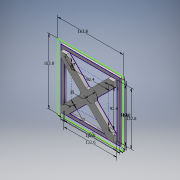
# Autodesk Inventor part: Lifting Motor Platform
Saved by Autodesk Inventor 2016 (Build 200138000, 138)
## iProperties
Created: 2016-03-08
Part Number: Lifting Motor Platform
Material: Generic
Document SubType Name: Modeling
Designer: Kenneth Daniel
Density: 1 g/cm^3
Appearance: Default
Author: Kenneth Daniel
Autodesk Inventor part; units mm, degrees
note: some values were not read from the file. Chosen so that the rebuilt part matches the saved one: sketch regions of "Extrusion5".
ref_plane "YZ Plane" through (0, 0, 0) normal (1, 0, 0) x (0, 1, 0)
ref_plane "XZ Plane" through (0, 0, 0) normal (0, 1, 0) x (-1, 0, 0)
ref_plane "XY Plane" through (0, 0, 0) normal (0, 0, 1) x (1, 0, 0)
sketch "Sketch1" plane through (0, 0, 0) normal (0, 1, 0) x (-1, 0, 0)
  line L0 (-81.5, 81.5) -> (81.5, -81.5) construction
  line L1 (-81.5, -81.5) -> (81.5, 81.5) construction
  line L2 (-66.3, 66.3) -> (66.3, -66.3) construction
  line L3 (-66.3, -66.3) -> (66.3, 66.3) construction
  line L4 (-81.9, 81.9) -> (-81.9, -81.9)
  line L5 (-81.9, -81.9) -> (81.9, -81.9)
  line L6 (81.9, -81.9) -> (81.9, 81.9)
  line L7 (81.9, 81.9) -> (-81.9, 81.9)
  line L8 (-66.1, 66.1) -> (-66.1, -66.1)
  line L9 (-66.1, -66.1) -> (66.1, -66.1)
  line L10 (66.1, -66.1) -> (66.1, 66.1)
  line L11 (66.1, 66.1) -> (-66.1, 66.1)
  line L12 (-66.1, 66.1) -> (66.1, -66.1) construction
  line L13 (-66.1, -66.1) -> (66.1, 66.1) construction
  line L14 (66.1, 51.9579) -> (17.2261, 3.084)
  line L15 (51.9579, 66.1) -> (3.084, 17.2261)
  line L16 (66.1, -51.9579) -> (14.1421, 0) construction
  line L17 (50.106, -64.2481) -> (3.084, -17.2261)
  arc A0 (-17.2261, -3.084) -> (-3.084, -17.2261) centre (0, 0) ccw
  arc A1 (-17.2261, 3.084) -> (-17.2261, -3.084) centre (0, 0) ccw
  line L18 (-14.1421, 0) -> (-17.2261, -3.084) construction
  line L19 (-3.084, 17.2261) -> (-51.9579, 66.1)
  line L20 (3.084, 17.2261) -> (0, 14.1421) construction
  line L21 (0, 14.1421) -> (-14.1421, 0) construction
  line L22 (14.1421, 0) -> (-3.084, 17.2261) construction
  arc A2 (17.2261, 3.084) -> (-17.2261, 3.084) centre (0, 0) ccw
  arc A3 (17.2261, -3.084) -> (17.2261, 3.084) centre (0, 0) ccw
  arc A4 (-3.084, -17.2261) -> (17.2261, -3.084) centre (0, 0) ccw
  line L23 (3.084, -17.2261) -> (0, -14.1421) construction
  line L24 (0, -14.1421) -> (-14.1421, 0) construction
  line L25 (17.2261, 3.084) -> (-3.084, -17.2261) construction
  line L26 (-3.084, -17.2261) -> (-51.9579, -66.1)
  line L27 (-17.2261, -3.084) -> (-66.1, -51.9579)
  line L28 (-17.2261, 3.084) -> (-64.2481, 50.106)
  line L29 (-14.1421, 0) -> (-17.2261, 3.084) construction
  line L30 (17.2261, -3.084) -> (66.1, -51.9579)
  line L31 (50.106, -64.2481) -> (51.9579, -66.1)
  line L32 (-64.2481, 50.106) -> (-66.1, 51.9579)
  line L33 (46.2, 46.2) -> (-46.2, 46.2) construction
  line L34 (-46.2, 46.2) -> (-46.2, -46.2) construction
  line L35 (-46.2, -46.2) -> (46.2, -46.2) construction
  line L36 (46.2, -46.2) -> (46.2, 46.2) construction
  line L37 (46.2, 46.2) -> (-46.2, -46.2) construction
  line L38 (-46.2, 46.2) -> (46.2, -46.2) construction
  circle A5 centre (46.2, -46.2) radius 1
  circle A6 centre (-46.2, -46.2) radius 1
  circle A7 centre (-46.2, 46.2) radius 1
  circle A8 centre (46.2, 46.2) radius 1
  line L39 (51.9579, 66.1) -> (66.1, 51.9579)
  line L40 (66.1, -51.9579) -> (51.9579, -66.1)
  line L41 (-51.9579, -66.1) -> (-66.1, -51.9579)
  line L42 (-66.1, 51.9579) -> (-51.9579, 66.1)
  line L43 (-74, 74) -> (-74, -74)
  line L44 (-74, -74) -> (74, -74)
  line L45 (74, -74) -> (74, 74)
  line L46 (74, 74) -> (-74, 74)
  line L47 (-74, 74) -> (74, -74) construction
  line L48 (-74, -74) -> (74, 74) construction
  dimension "d0" = 163
  dimension "d1" = 163
  dimension "d2" = 132.6
  dimension "d3" = 132.6
  dimension "d5" = 163.8
  dimension "d6" = 163.8
  dimension "d7" = 132.2
  dimension "d8" = 132.2
  dimension "d9" = 20
  dimension "d10" = 20
  dimension "d11" = 35
  dimension "d12" = 92.4
  dimension "d13" = 92.4
  dimension "d14" = 2
  dimension "d15" = 2
  dimension "d16" = 2
  dimension "d17" = 2
  dimension "d28" = 148
  dimension "d29" = 148
  constraints: 98 end point, 41 parallel, 23 point on line, 15 point on circle, 10 midpoint, 9 centre point, 7 perpendicular, 5 coincident, 2 vertical, 1 collinear, 1 horizontal, 2 other
  measures "d0" distance of L0.start L1.start
  measures "d1" distance of L0.end L1.start
  measures "d2" distance of L2.start L3.start
  measures "d3" distance of L2.end L3.start
  measures "d5" distance of L6.end L4.start
  measures "d6" distance of L5.end L6.end
  measures "d7" distance of L8.start L8.end
  measures "d8" distance of L9.end L8.end
  measures "d9" distance between parallel lines of L15 L14
  measures "d10" distance between parallel lines of L17 L16
  measures "d11" diameter of A0
  measures "d12" distance of L33.start L33.end
  measures "d13" distance of L34.end L33.end
  measures "d14" diameter of A5
  measures "d15" diameter of A6
  measures "d16" diameter of A7
  measures "d17" diameter of A8
  measures "d28" distance of L43.start L43.end
  measures "d29" distance of L44.end L43.end
extrude "Extrusion1" add sketch "Sketch1" along normal blind 5 contours L7 L6 L5 L4 | L46 L45 L44 L43
extrude "Extrusion2" add sketch "Sketch1" along normal blind 5 contours L11 L42 L8 | L41 L9 L8 | L11 L10 L39 | L40 L10 L9
extrude "Extrusion4" cut sketch "Sketch1" against normal blind 10 contours L11 L42 L8 | L42 L19 A2 L28 L32 | L41 L9 L8 | L27 A0 L26 L41 | L39 L14 A2 L15 | L11 L10 L39 | A2 A3 A4 A0 A1 | L40 L10 L9 | L31 L17 A4 L30 L40 | A7
extrude "Extrusion5" add sketch "Sketch1" against normal blind 8 contours L11 L42 L8 | L42 L19 A2 L28 L32 | L41 L9 L8 | L27 A0 L26 L41 | L39 L14 A2 L15 | L11 L10 L39 | A2 A3 A4 A0 A1 | L40 L10 L9 | L31 L17 A4 L30 L40
extrude "Extrusion6" cut sketch "Sketch1" along normal blind 8 contours L7 L6 L5 L4
body "Solid1"
